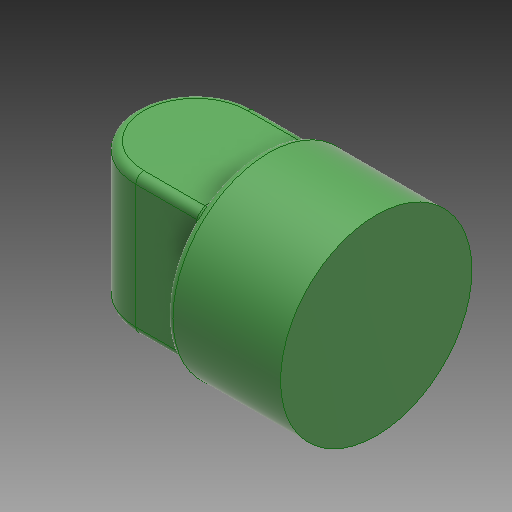
# Autodesk Inventor part: SimplifiedThigh
Saved by Autodesk Inventor 2018 (Build 220112000, 112)
## iProperties
Part Number: SimplifiedThigh
Material: Generisch
Document SubType Name: Modeling
Designer: Jochen Alt
Mass: 81.7563 g
Surface Area: 111.027 cm^2
Volume: 81.7563 cm^3
Density: 1 g/cm^3
Appearance: Glatt - waldgrün
Author: Jochen Alt
Autodesk Inventor part; units mm, degrees
ref_plane "YZ Plane" through (0, 0, 0) normal (1, 0, 0) x (0, 1, 0)
ref_plane "XZ Plane" through (0, 0, 0) normal (0, 1, 0) x (-1, 0, 0)
ref_plane "XY Plane" through (0, 0, 0) normal (0, 0, 1) x (1, 0, 0)
sketch "Skizze Servo Projektion" plane through (0, 0, 0) normal (0, 0, 1) x (1, 0, 0)
  circle A0 centre (6.3, 9) radius 0.85 construction
  circle A1 centre (6.3, -9) radius 0.85 construction
  circle A2 centre (-32.7, -9) radius 0.85 construction
  circle A3 centre (-32.7, 9) radius 0.85 construction
  circle A4 centre (-26.0282, 0) radius 9.5 construction
  line L0 (0.03, 10) -> (0.03, 11.5) construction
  arc A5 (0.03, 10) -> (1.9, 8.13) centre (1.9, 10) ccw construction
  line L1 (3.3264, 8.13) -> (1.9, 8.13) construction
  arc A6 (3.8197, 7.7121) -> (3.3264, 8.13) centre (3.3264, 7.63) ccw construction
  arc A7 (3.8197, 7.7121) -> (5.25, 6.5) centre (5.25, 7.95) ccw construction
  line L2 (5.25, 6.5) -> (9, 6.5) construction
  line L3 (9, 8.0017) -> (9, 6.5) construction
  arc A8 (9.0005, 8.0017) -> (5.3017, 11.7005) centre (5.3, 8) ccw construction
  line L4 (3.75, 11.7) -> (5.3017, 11.7) construction
  line L5 (3.75, 11.7) -> (3.75, 10.9) construction
  line L6 (3.75, 10.9) -> (3.4008, 10.9) construction
  arc A9 (1.15, 11.5811) -> (3.4008, 10.9) centre (1.9, 10) ccw construction
  line L7 (1.15, 11.7) -> (1.15, 11.5811) construction
  line L8 (-0.0117, 11.7) -> (1.15, 11.7) construction
  arc A10 (0.03, 11.5) -> (-0.0117, 11.7) centre (-0.47, 11.5) ccw construction
  arc A11 (6.3002, 10.3002) -> (6.3, 7.6998) centre (6.3, 9) ccw construction
  arc A12 (6.3, 7.6996) -> (6.3002, 10.3004) centre (6.3, 9) ccw construction
  line L9 (-0.0117, -11.7) -> (1.15, -11.7) construction
  line L10 (1.15, -11.7) -> (1.15, -11.5811) construction
  arc A13 (3.4008, -10.9) -> (1.15, -11.5811) centre (1.9, -10) ccw construction
  line L11 (3.75, -10.9) -> (3.4008, -10.9) construction
  line L12 (3.75, -11.7) -> (3.75, -10.9) construction
  line L13 (5.3017, -11.7) -> (3.75, -11.7) construction
  arc A14 (5.3017, -11.7005) -> (9.0005, -8.0017) centre (5.3, -8) ccw construction
  line L14 (9, -6.5) -> (9, -8.0017) construction
  line L15 (9, -6.5) -> (5.25, -6.5) construction
  arc A15 (5.25, -6.5) -> (3.8197, -7.7121) centre (5.25, -7.95) ccw construction
  arc A16 (3.3264, -8.13) -> (3.8197, -7.7121) centre (3.3264, -7.63) ccw construction
  line L16 (3.3264, -8.13) -> (1.9, -8.13) construction
  arc A17 (1.9, -8.13) -> (0.03, -10) centre (1.9, -10) ccw construction
  line L17 (0.03, -10) -> (0.03, -11.5) construction
  arc A18 (-0.0117, -11.7) -> (0.03, -11.5) centre (-0.47, -11.5) ccw construction
  arc A19 (6.2998, -7.6997) -> (6.3, -10.3003) centre (6.3, -9) ccw construction
  arc A20 (6.3, -10.3002) -> (6.2998, -7.6998) centre (6.3, -9) ccw construction
  line L18 (-34.4734, 6.5) -> (-34.4734, 6.702) construction
  line L19 (-30.9117, 6.702) -> (-34.4734, 6.702) construction
  arc A21 (-30.9117, 6.702) -> (-30.2197, 7.7121) centre (-31.65, 7.95) ccw construction
  arc A22 (-29.7264, 8.13) -> (-30.2197, 7.7121) centre (-29.7264, 7.63) ccw construction
  line L20 (-29.7264, 8.13) -> (-28.3, 8.13) construction
  arc A23 (-28.3, 8.13) -> (-26.43, 10) centre (-28.3, 10) ccw construction
  line L21 (-26.43, 11.7) -> (-26.43, 10) construction
  line L22 (-27.55, 11.7) -> (-26.43, 11.7) construction
  line L23 (-27.55, 11.7) -> (-27.55, 11.5811) construction
  arc A24 (-29.8008, 10.9) -> (-27.55, 11.5811) centre (-28.3, 10) ccw construction
  line L24 (-30.15, 10.9) -> (-29.8008, 10.9) construction
  line L25 (-30.15, 11.7) -> (-30.15, 10.9) construction
  line L26 (-31.7017, 11.7) -> (-30.15, 11.7) construction
  arc A25 (-31.7017, 11.7005) -> (-35.4005, 8.0017) centre (-31.7, 8) ccw construction
  line L27 (-35.4, 6.5) -> (-35.4, 8.0017) construction
  line L28 (-35.4, 6.5) -> (-34.4734, 6.5) construction
  circle A26 centre (-32.7, 9) radius 1.3004 construction
  line L29 (-30.4301, -7.1662) -> (-34.4734, -7.1662) construction
  line L30 (-34.4734, -6.5) -> (-34.4734, -7.1662) construction
  line L31 (-34.4734, -6.5) -> (-35.4, -6.5) construction
  line L32 (-35.4, -8.0012) -> (-35.4, -6.5) construction
  arc A27 (-35.4005, -8.0012) -> (-31.7017, -11.7005) centre (-31.7, -8) ccw construction
  line L33 (-30.15, -11.7) -> (-31.7017, -11.7) construction
  line L34 (-30.15, -11.7) -> (-30.15, -10.9) construction
  line L35 (-30.15, -10.9) -> (-29.8008, -10.9) construction
  arc A28 (-27.55, -11.5811) -> (-29.8008, -10.9) centre (-28.3, -10) ccw construction
  line L36 (-27.55, -11.7) -> (-27.55, -11.5811) construction
  line L37 (-26.43, -11.7) -> (-27.55, -11.7) construction
  line L38 (-26.43, -11.7) -> (-26.43, -10) construction
  arc A29 (-26.43, -10) -> (-28.3, -8.13) centre (-28.3, -10) ccw construction
  line L39 (-29.7264, -8.13) -> (-28.3, -8.13) construction
  arc A30 (-30.2197, -7.7121) -> (-29.7264, -8.13) centre (-29.7264, -7.63) ccw construction
  arc A31 (-30.2197, -7.7121) -> (-30.4301, -7.1662) centre (-31.65, -7.95) ccw construction
  circle A32 centre (-32.7, -9) radius 1.3004 construction
  line L40 (-35.4, 8.0001) -> (-35.4, 6.5) construction
  arc A33 (-31.7001, 11.7) -> (-35.4, 8.0001) centre (-31.7, 8) ccw construction
  line L41 (-30.2, 11.7) -> (-31.7001, 11.7) construction
  line L42 (-30.2, 7.95) -> (-30.2, 11.7) construction
  arc A34 (-31.65, 6.5) -> (-30.2, 7.95) centre (-31.65, 7.95) ccw construction
  line L43 (-35.4, 6.5) -> (-31.65, 6.5) construction
  circle A35 centre (-32.7, 9) radius 1 construction
  line L44 (-31.7001, -11.7) -> (-30.2, -11.7) construction
  arc A36 (-35.4, -8.0001) -> (-31.7001, -11.7) centre (-31.7, -8) ccw construction
  line L45 (-35.4, -6.5) -> (-35.4, -8.0001) construction
  line L46 (-35.4, -6.5) -> (-31.65, -6.5) construction
  arc A37 (-30.2, -7.95) -> (-31.65, -6.5) centre (-31.65, -7.95) ccw construction
  line L47 (-30.2, -7.95) -> (-30.2, -11.7) construction
  circle A38 centre (-32.7, -9) radius 1 construction
  line L48 (3.8, -11.4999) -> (3.8, -7.95) construction
  arc A39 (5.25, -6.5) -> (3.8, -7.95) centre (5.25, -7.95) ccw construction
  line L49 (5.25, -6.5) -> (8.9886, -6.5) construction
  ellipse E0 centre (8.9925, -6.4605) end of major axis (8.8053, -6.4614) minor radius 0.0394 (8.9886, -6.5) -> (9, -6.4999) ccw construction
  line L50 (9, -8) -> (9, -6.4999) construction
  arc A40 (5.3, -11.7) -> (9, -8) centre (5.3, -8) ccw construction
  line L51 (3.7582, -11.7) -> (5.3, -11.7) construction
  arc A41 (3.7582, -11.7) -> (3.8, -11.4999) centre (3.2999, -11.4999) ccw construction
  circle A42 centre (6.3, -9) radius 1 construction
  line L52 (3.7582, 11.7) -> (5.3, 11.7) construction
  arc A43 (9, 8) -> (5.3, 11.7) centre (5.3, 8) ccw construction
  line L53 (9, 6.4999) -> (9, 8) construction
  ellipse E1 centre (8.9925, 6.4605) end of major axis (8.8053, 6.4614) minor radius 0.0394 (9, 6.4999) -> (8.9886, 6.5) ccw construction
  line L54 (5.25, 6.5) -> (8.9886, 6.5) construction
  arc A44 (3.8, 7.95) -> (5.25, 6.5) centre (5.25, 7.95) ccw construction
  line L55 (3.8, 11.4999) -> (3.8, 7.95) construction
  arc A45 (3.8, 11.4999) -> (3.7582, 11.7) centre (3.2999, 11.4999) ccw construction
  circle A46 centre (6.3, 9) radius 1 construction
  line L56 (-14.1, 10.2) -> (-14.1, -10.2) construction
  line L57 (-9.1, -10.2) -> (-9.1, 10.2) construction
  line L58 (-3.4016, 1.5) -> (3.0621, 1.5) construction
  ellipse E2 centre (-3.3983, 1.8017) end of major axis (-3.6128, 1.5872) minor radius 0.3 (-3.7, 1.7984) -> (-3.4016, 1.5) ccw construction
  line L59 (-3.7, 2.5) -> (-3.7, 1.7984) construction
  line L60 (-8.6653, 4.1133) -> (-3.7, 2.5) construction
  ellipse E3 centre (-8.4844, 4.5832) end of major axis (-9.0452, 4.6462) minor radius 0.5 (-9.048, 4.5967) -> (-8.6653, 4.1133) ccw construction
  line L61 (-9.048, -4.5967) -> (-9.048, 4.5967) construction
  ellipse E4 centre (-8.4844, -4.5832) end of major axis (-9.0452, -4.6462) minor radius 0.5 (-8.6653, -4.1133) -> (-9.048, -4.5967) ccw construction
  line L62 (-3.7, -2.5) -> (-8.6653, -4.1133) construction
  line L63 (-3.7, -2.5) -> (-3.7, -1.7984) construction
  ellipse E5 centre (-3.3983, -1.8017) end of major axis (-3.6128, -1.5872) minor radius 0.3 (-3.4016, -1.5) -> (-3.7, -1.7984) ccw construction
  line L64 (-3.4016, -1.5) -> (3.0621, -1.5) construction
  ellipse E6 centre (3.0403, -3.5108) end of major axis (1.6076, -4.9373) minor radius 1.9999 (4.5504, -2.1667) -> (3.0621, -1.5) ccw construction
  ellipse E7 centre (5.3055, -1.4945) end of major axis (4.5906, -2.2094) minor radius 1 (4.5504, -2.1667) -> (5.2945, -2.5) ccw construction
  line L65 (9, -2.5) -> (5.2945, -2.5) construction
  line L66 (9, 2.5) -> (9, -2.5) construction
  line L67 (9, 2.5) -> (5.2945, 2.5) construction
  ellipse E8 centre (5.3055, 1.4945) end of major axis (4.5906, 2.2094) minor radius 1 (5.2945, 2.5) -> (4.5504, 2.1667) ccw construction
  ellipse E9 centre (3.0403, 3.5108) end of major axis (1.6077, 4.9373) minor radius 1.9999 (3.0621, 1.5) -> (4.5504, 2.1667) ccw construction
  circle A47 centre (0, 0) radius 1 construction
  line L68 (-7.0181, -1.8024) -> (-7.0181, -1.25) construction
  arc A48 (-7.0181, 1.7382) -> (-7.0181, -1.8024) centre (-7.1503, -0.0321) ccw construction
  line L69 (-7.0181, 1.1858) -> (-7.0181, 1.7382) construction
  arc A49 (-7.0181, 1.1858) -> (-7.0181, -1.25) centre (-7.1503, -0.0321) ccw construction
  line L70 (-4.4623, -0.3083) -> (-4.4623, 0.2441) construction
  line L71 (-5.409, -0.3083) -> (-4.4623, -0.3083) construction
  arc A50 (-5.409, -0.3083) -> (-4.0833, -1.25) centre (-4.2155, -0.0321) ccw construction
  line L72 (-4.0833, -1.8024) -> (-4.0833, -1.25) construction
  arc A51 (-4.0833, 1.7382) -> (-4.0833, -1.8024) centre (-4.2155, -0.0321) ccw construction
  line L73 (-4.0833, 1.1858) -> (-4.0833, 1.7382) construction
  arc A52 (-4.0833, 1.1858) -> (-5.409, 0.2441) centre (-4.2155, -0.0321) ccw construction
  line L74 (-4.4623, 0.2441) -> (-5.409, 0.2441) construction
  line L75 (-13.7722, 12) -> (-9.4278, 12) construction
  line L76 (-9.4278, -12) -> (-13.7722, -12) construction
  line L77 (9.3, 2.7701) -> (9.3, -2.7701) construction
  line L78 (-35.7, -6.2) -> (-35.7, 6.2) construction
  arc A53 (-31.7001, 12) -> (-35.7, 8.0001) centre (-31.7, 8) ccw construction
  arc A54 (9.3, 8.0001) -> (5.3001, 12) centre (5.3, 8) ccw construction
  arc A55 (5.3001, -12) -> (9.3, -8.0001) centre (5.3, -8) ccw construction
  arc A56 (-35.7, -8.0001) -> (-31.7001, -12) centre (-31.7, -8) ccw construction
  line L79 (-26.0282, 15) -> (11.3, 15)
  line L80 (11.3, 15) -> (11.3, -15)
  line L81 (11.3, -15) -> (-26.0282, -15)
  line L82 (18.4014, 0) -> (11.3, 0) construction
  line L83 (0, 0) -> (-45.3062, 0) construction
  arc A57 (-26.0282, 15) -> (-26.0282, -15) centre (-26.0282, 0) ccw
  line L84 (18.4014, 0) -> (-45.3062, 0) construction
  line L85 (18.4014, 0) -> (-45.3062, 0) construction
  line L86 (0, -17.8457) -> (0, 16.9839) construction
  line L87 (11.3, 15) -> (19.3, 15)
  line L88 (19.3, 15) -> (19.3, -15)
  line L89 (19.3, -15) -> (11.3, -15)
  line L90 (11.3, -15) -> (11.3, 15)
  dimension "d4" = 2
  dimension "d5" = 15
  dimension "d121" = 8
  constraints: 24 end point, 6 horizontal, 3 parallel, 2 perpendicular, 2 point on circle, 2 tangent, 1 centre point, 1 coincident, 1 midpoint, 1 vertical, 18 other
  measures "d4" distance between parallel lines of L80 L77
  measures "d5" radius of A57
  measures "d121" distance of L88.end L89.end
ref_plane "Arbeitsebene1" through (11.3, -15, 0) normal (1, 0, 0) x (0, 0, -1)
extrude "Extrusion3" add sketch "Skizze Servo Projektion" against normal blind 35
sketch "Skizze2" plane through (11.3, -15, 0) normal (1, 0, 0) x (0, 0, -1)
  line L0 (35, 30) -> (35, 0) projected
  circle A0 centre (17.5, 15) radius 24
  point P0 (0, 15)
  constraints: 1 centre point
extrude "Extrusion2" add sketch "Skizze2" against normal blind 21 and the other way blind 8
ref_plane "Arbeitsebene2" through (0, 0, -2.5) normal (0, 0, 1) x (1, 0, 0)
ref_plane "Arbeitsebene6" through (0, 0, 0) normal (0, 0, 1) x (1, 0, 0)
ref_plane "Arbeitsebene7" through (0, 0, -17.5) normal (0, 0, 1) x (1, 0, 0)
fillet "Rundung1" radius 2 6 edges at (-41.0282, 0, 0) (-17.8641, 15, 0) (-17.8641, -15, 0) (-41.0282, 0, -35) (-17.8641, 15, -35) (-17.8641, -15, -35)
fillet "Rundung7" radius 2 1 edges at (-9.7, 0, 6.5)
fillet "Rundung8" radius 1 12 edges at (-9.7, 14.9666, -33.3641) (-9.6867, 14.2853, -34.5324) (-9.7, 0, -35) (-9.7, -14.9666, -33.3641) (-9.6867, -14.2852, -34.5324) (-9.7, -15, -17.5) (-9.7, -14.9666, -1.6359) (-9.6867, -14.2853, -0.4676) (-9.7, 0, 0) (-9.7, 14.9666, -1.6359) (-9.6867, 14.2852, -0.4676) (-9.7, 15, -17.5)
